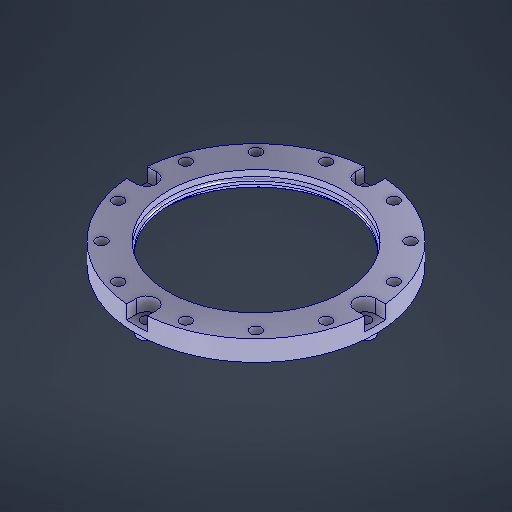
# Autodesk Inventor part: CR_OUTSIDE,TOP,REV-ENG
Saved by Autodesk Inventor 2026.2 (Build 302298010, 298A)
## iProperties
Created: 2026-03-05
Part Number: CR_OUTSIDE,TOP,REV-ENG
Material: Stainless Steel, 316L
Document SubType Name: Modeling
Designer: 4aida
Density: 8 g/cm^3
Appearance: Blue Chrome
Author: 4aida
Autodesk Inventor part; units mm, degrees
ref_plane "YZ Plane" through (0, 0, 0) normal (1, 0, 0) x (0, 1, 0)
ref_plane "XZ Plane" through (0, 0, 0) normal (0, 1, 0) x (-1, 0, 0)
ref_plane "XY Plane" through (0, 0, 0) normal (0, 0, 1) x (1, 0, 0)
sketch "Sketch1" plane through (0, 0, 0) normal (1, 0, 0) x (0, 1, 0)
  line L0 (-4.2955, 0) -> (4.2955, 0)
  line L1 (0, 35) -> (0, 28.0784) construction
  line L2 (-2.5784, 25.25) -> (-3, 25.25) construction
  line L3 (-3, 25.25) -> (-3, 35) construction
  line L4 (-3, 35) -> (0, 35) construction
  line L5 (-2.5784, 25.25) -> (-0.25, 27.5784) construction
  line L6 (-0.25, 27.5784) -> (-0.25, 28.0784) construction
  line L7 (-0.25, 28.0784) -> (0, 28.0784) construction
  line L8 (0, 22.1716) -> (-2.8284, 25) construction
  line L9 (-2.8284, 25) -> (0, 27.8284) construction
  line L10 (0, 27.8284) -> (2.8284, 25) construction
  line L11 (2.8284, 25) -> (0, 22.1716) construction
  line L12 (0, 22.1716) -> (0, 27.8284) construction
  line L13 (-2.8284, 25) -> (2.8284, 25) construction
  line L14 (0, 28.0784) -> (0, 35)
  line L15 (0, 35) -> (6, 35)
  line L16 (6, 35) -> (6, 25.6875)
  line L17 (6, 25.6875) -> (4.25, 25.6875)
  arc A0 (4.25, 25.6875) -> (3.4232, 25.25) centre (4.25, 24.6875) ccw
  line L18 (3.4232, 25.25) -> (2.5784, 25.25)
  line L19 (2.5784, 25.25) -> (0.25, 27.5784)
  line L20 (0.25, 27.5784) -> (0.25, 28.0784)
  line L21 (0.25, 28.0784) -> (0, 28.0784)
  circle A1 centre (4.25, 24.6875) radius 1 construction
  point P0 (0, 0)
  point P1 (0, 0)
  point P2 (0, 0)
  point P3 (0, 25)
  point P4 (-1.4142, 26.4142)
  dimension "d0" = 3
  dimension "d1" = 0.5
  dimension "d2" = 0.25
  dimension "d3" = 135
  dimension "d4" = 4
  dimension "d5" = 50
  dimension "d6" = 0.25
  dimension "d7" = 70
  dimension "d8" = 0.25
  dimension "d9" = 2
  dimension "d10" = 0.3125
  dimension "d12" = 6
  dimension "d13" = 4.25
  constraints: 44 end point, 10 perpendicular, 5 midpoint, 4 point on circle, 3 horizontal, 3 point on line, 3 vertical, 2 centre point, 2 coincident, 2 parallel, 2 tangent, 1 collinear, 1 horizontal alignment, 1 vertical alignment
  measures "d0" distance between parallel lines of L3 L1
  measures "d1" distance of L5.end L6.end
  measures "d2" distance of L6.end L7.end
  measures "d3" angle of L2 L5
  measures "d4" distance of L12.end L11.start
  measures "d5" diameter of L11.start L0
  measures "d6" distance from line of L8.end L2
  measures "d7" diameter of L4 L0
  measures "d8" distance of L20.end L7.end
  measures "d9" diameter of A1
  measures "d10" vertical distance of A1.centre L11.start
  measures "d12" distance between parallel lines of L1 L16
  measures "d13" horizontal distance of A1.centre point (0, 25)
revolve "Revolution1" add sketch "Sketch1" angle 360 about axis through (0, -4.2955, 0) along (0, 1, 0)
sketch "Sketch5" plane through (0, 0, 0) normal (0, -1, 0) x (1, 0, 0)
  circle A0 centre (0, 32) radius 2.5
  line L0 (0, 0) -> (0, 35) construction
  circle A1 centre (0, 0) radius 35 construction
  circle A2 centre (-32, 0) radius 2.5
  circle A3 centre (0, -32) radius 2.5
  circle A4 centre (32, 0) radius 2.5
  dimension "d45" = 3
  dimension "d46" = 5
  dimension "d49" = 360
  constraints: 4 centre point, 2 end point, 1 point on line, 1 vertical, 1 vertical alignment, 10 other
  measures "d45" distance of A0.centre L0.end
  measures "d46" diameter of A0
extrude "Extrusion2" add sketch "Sketch5" along normal blind 1.5
sketch "Sketch2" plane through (0, 6, 0) normal (0, 1, 0) x (1, 0, 0)
  circle A0 centre (0, 0) radius 35 construction
  circle A1 centre (0, -32) radius 3 construction
  circle A2 centre (0, 0) radius 35 construction
  line L0 (0, 0) -> (0, -35)
  point P0 (0, 0)
  dimension "d43" = 3
  constraints: 3 vertical alignment, 2 end point, 1 centre point, 1 coincident, 3 other
  measures "d43" distance of L0.end point (0, -32)
hole "Hole1" at (0, 6, 32) direction (0, -1, 0) diameter 3.2 end through all counterbore diameter 6 counterbore depth 4 clearance for "Socket Head Cap Screw" size "M3" standard "Ansi Metric M Profile"
sketch "Sketch3" plane through (0, 6, 0) normal (0, 1, 0) x (-1, 0, 0)
  circle A0 centre (0, 32) radius 3 projected
  circle A1 centre (0, 0) radius 35 projected
  circle A2 centre (0, 0) radius 25.6875 projected
  circle A3 centre (0, 32) radius 3 projected
  circle A4 centre (0, 0) radius 35 projected
  line L0 (3, 32) -> (3, 34.8712)
  line L1 (-3, 32) -> (-3, 34.8712)
  point P0 (0, 0)
  point P1 (0, 35)
  point P2 (-3, 34.8712)
  point P3 (3, 34.8712)
  point P4 (0, 35)
  constraints: 4 end point, 4 point on circle, 4 tangent, 1 parallel, 1 vertical
extrude "Extrusion1" cut sketch "Sketch3" against normal up to surface (4 mm away) contours L1 A1 A0 | A0 A1 L0
pattern_circular "Circular Pattern1" count 4 over 360 about axis through (0, 3, 0) along (0, 1, 0) of "Hole1", "Extrusion1"
sketch "Sketch4" plane through (0, 6, 32) normal (0, 1, 0) x (1, 0, 0)
  arc A0 (3, -2.8712) -> (34.8712, 29) centre (0, 32) ccw construction
  circle A1 centre (-9.8885, 1.5662) radius 3 construction
  circle A2 centre (0, 0) radius 1.6 construction
  line L0 (0, 0) -> (0, 32) construction
  line L1 (0, 32) -> (-9.8885, 1.5662) construction
  point P0 (-27.8388, 22.1642)
  dimension "d27" = 18
  dimension "d44" = 6
  constraints: 4 end point, 1 centre point, 1 coincident, 1 tangent, 1 vertical
  measures "d27" angle of L1 L0
  measures "d44" diameter of A1
hole "Hole2" at (-9.8885, 6, 30.4338) direction (0, -1, 0) diameter 3.242 end through all thread size "M4x0.7" class "6H" standard "ANSI Metric M Profile"
pattern_circular "Circular Pattern2" count 3 over 54 about axis through (0, 3, 0) along (0, -1, 0) of "Hole2"
pattern_circular "Circular Pattern3" count 4 over 360 about axis through (0, 3, 0) along (0, 1, 0) of "Hole2", "Circular Pattern2"
equation "\"d2\" = 0.5 * d1"
equation "\"d8\" = d2"
body "Solid1"
